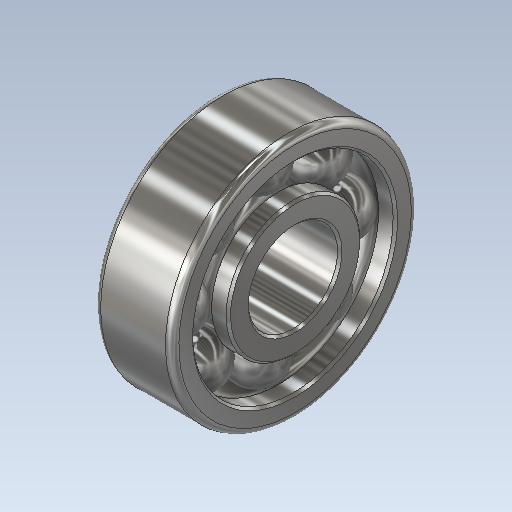
# Autodesk Inventor part: ROLAMENTO_608Z
Saved by Autodesk Inventor 2020.2 (Build 242310000, 310)
## iProperties
Created: 2017-03-31
Part Number: ROLAMENTO_608Z
Material: Generic
Document SubType Name: Modeling
Designer: Richard
Density: 1 g/cm^3
Appearance: Chrome - Polished
Author: Richard
Autodesk Inventor part; units mm, degrees
ref_plane "YZ Plane" through (0, 0, 0) normal (1, 0, 0) x (0, 1, 0)
ref_plane "XZ Plane" through (0, 0, 0) normal (0, 1, 0) x (-1, 0, 0)
ref_plane "XY Plane" through (0, 0, 0) normal (0, 0, 1) x (1, 0, 0)
sketch "Sketch1" plane through (0, 0, 0) normal (1, 0, 0) x (0, 1, 0)
  point P0 (0, 0)
sketch "Sketch2" plane through (0, 0, 0) normal (0, 0, 1) x (1, 0, 0)
  line L0 (-3.5, -7.4748) -> (3.5, -7.4748)
  line L1 (2.9, 3.5252) -> (-2.9, 3.5252)
  line L2 (-3.5, -3.4748) -> (3.5, -3.4748)
  arc A0 (-2.9, 3.5252) -> (-3.5, 2.9252) centre (-2.9, 2.9252) ccw
  arc A1 (3.5, 2.9252) -> (2.9, 3.5252) centre (2.9, 2.9252) ccw
  line L3 (3.5, -3.4748) -> (3.5, -1.5)
  line L4 (3.5, 1.5) -> (3.5, 2.9252)
  line L5 (-3.5, 2.9252) -> (-3.5, 1.5)
  line L6 (-3.5, -1.5) -> (-3.5, -3.4748)
  arc A2 (-2, -1.5) -> (2, -1.5) centre (0, 0) ccw
  arc A3 (2, 1.5) -> (-2, 1.5) centre (0, 0) ccw
  line L7 (-3.5, 1.5) -> (-2, 1.5)
  line L8 (2, 1.5) -> (3.5, 1.5)
  line L9 (-3.5, -1.5) -> (-2, -1.5)
  line L10 (2, -1.5) -> (3.5, -1.5)
  point P0 (-3.5, 3.5252)
  dimension "d7" = 4
  dimension "d8" = 11
  dimension "d9" = 0.6
  constraints: 22 end point, 8 point on circle, 7 parallel, 6 tangent, 4 centre point, 2 perpendicular, 1 coincident, 1 equal radius, 1 horizontal, 1 point on line
  measures "d7" distance between parallel lines of L2 L0
  measures "d8" distance of point (-3.5, 3.525) L0.start
  measures "d9" radius of A0
revolve "Revolution1" add sketch "Sketch2" angle 360 about axis through (-3.5, -7.4748, 0) along (1, 0, 0)
sketch "Sketch3" plane through (0, 0, 0) normal (0, 0, 1) x (1, 0, 0)
  arc A0 (0, 2.4) -> (0, -2.4) centre (0, 0) ccw
  line L0 (0, 2.4) -> (0, -2.4)
  dimension "d11" = 4.8
  constraints: 2 end point, 2 point on circle, 1 centre point, 1 coincident, 1 vertical
  measures "d11" diameter of A0
revolve "Revolution2" add sketch "Sketch3" angle 360 about axis through (0, 2.4, 0) along (0, -1, 0)
pattern_circular "Circular Pattern1" count 8 over 360 about axis through (0, -7.4748, 0) along (1, 0, 0) of "Revolution2"
chamfer "Chamfer1" distance 0.2 angle 45 1 edges at (3.5, -11.4748, 0)
chamfer "Chamfer2" distance 0.2 angle 45 1 edges at (3.5, -16.4496, 0)
chamfer "Chamfer3" distance 0.2 angle 45 1 edges at (3.5, -13.4496, 0)
chamfer "Chamfer4" distance 0.2 angle 45 3 edges at (-3.5, -11.4748, 0) (-3.5, -16.4496, 0) (-3.5, -13.4496, 0)
body "Solid1"
